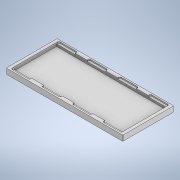
# Autodesk Inventor part: kbbottombodyethan
Saved by Autodesk Inventor 2021 (Build 250183000, 183)
## iProperties
Created: 2023-05-21
Part Number: kbbottombodyethan
Material: Generic
Document SubType Name: Modeling
Designer: ryand
Density: 1 g/cm^3
Appearance: Default
Author: ryand
Autodesk Inventor part; units mm, degrees
ref_plane "YZ Plane" through (0, 0, 0) normal (1, 0, 0) x (0, 1, 0)
ref_plane "XZ Plane" through (0, 0, 0) normal (0, 1, 0) x (-1, 0, 0)
ref_plane "XY Plane" through (0, 0, 0) normal (0, 0, 1) x (1, 0, 0)
sketch "Sketch1" plane through (0, 0, 0) normal (0, 1, 0) x (-1, 0, 0)
  line L0 (183.8315, -67.9127) -> (183.8315, 67.9127) construction
  line L1 (-179.8315, 79.4127) -> (-126.5543, 79.4127) construction
  line L2 (-122.5543, 75.4127) -> (-122.5543, 71.9127) construction
  line L3 (-81.7029, 71.9127) -> (-81.7029, 75.4127) construction
  line L4 (-77.7029, 79.4127) -> (-24.4257, 79.4127) construction
  line L5 (-20.4257, 75.4127) -> (-20.4257, 71.9127) construction
  line L6 (20.4257, 71.9127) -> (20.4257, 75.4127) construction
  line L7 (24.4257, 79.4127) -> (77.7029, 79.4127) construction
  line L8 (81.7029, 75.4127) -> (81.7029, 71.9127) construction
  line L9 (122.5543, 71.9127) -> (122.5543, 75.4127) construction
  line L10 (126.5543, 79.4127) -> (179.8315, 79.4127) construction
  line L11 (183.8315, 75.4127) -> (183.8315, 71.9127) construction
  line L12 (-126.5543, -79.4127) -> (-179.8315, -79.4127) construction
  line L13 (-183.8315, -75.4127) -> (-183.8315, -71.9127) construction
  line L14 (-122.5543, -71.9127) -> (-122.5543, -75.4127) construction
  line L15 (-81.7029, -75.4127) -> (-81.7029, -71.9127) construction
  line L16 (-24.4257, -79.4127) -> (-77.7029, -79.4127) construction
  line L17 (-20.4257, -71.9127) -> (-20.4257, -75.4127) construction
  line L18 (20.4257, -75.4127) -> (20.4257, -71.9127) construction
  line L19 (77.7029, -79.4127) -> (24.4257, -79.4127) construction
  line L20 (81.7029, -71.9127) -> (81.7029, -75.4127) construction
  line L21 (122.5543, -75.4127) -> (122.5543, -71.9127) construction
  line L22 (179.8315, -79.4127) -> (126.5543, -79.4127) construction
  line L23 (183.8315, -71.9127) -> (183.8315, -75.4127) construction
  line L24 (-122.5543, -71.9127) -> (-81.7029, -71.9127) construction
  line L25 (-20.4257, -71.9127) -> (20.4257, -71.9127) construction
  line L26 (81.7029, -71.9127) -> (122.5543, -71.9127) construction
  arc A0 (-183.8315, -75.4127) -> (-179.8315, -79.4127) centre (-179.8315, -75.4127) ccw construction
  arc A1 (-126.5543, -79.4127) -> (-122.5543, -75.4127) centre (-126.5543, -75.4127) ccw construction
  arc A2 (-81.7029, -75.4127) -> (-77.7029, -79.4127) centre (-77.7029, -75.4127) ccw construction
  arc A3 (-24.4257, -79.4127) -> (-20.4257, -75.4127) centre (-24.4257, -75.4127) ccw construction
  arc A4 (20.4257, -75.4127) -> (24.4257, -79.4127) centre (24.4257, -75.4127) ccw construction
  arc A5 (77.7029, -79.4127) -> (81.7029, -75.4127) centre (77.7029, -75.4127) ccw construction
  arc A6 (122.5543, -75.4127) -> (126.5543, -79.4127) centre (126.5543, -75.4127) ccw construction
  arc A7 (179.8315, -79.4127) -> (183.8315, -75.4127) centre (179.8315, -75.4127) ccw construction
  line L27 (183.8315, -67.9127) -> (183.8315, -71.9127) construction
  arc A8 (-179.8315, 79.4127) -> (-183.8315, 75.4127) centre (-179.8315, 75.4127) ccw construction
  arc A9 (-122.5543, 75.4127) -> (-126.5543, 79.4127) centre (-126.5543, 75.4127) ccw construction
  line L28 (-81.7029, 71.9127) -> (-122.5543, 71.9127) construction
  line L29 (20.4257, 71.9127) -> (-20.4257, 71.9127) construction
  line L30 (122.5543, 71.9127) -> (81.7029, 71.9127) construction
  line L31 (183.8315, 71.9127) -> (183.8315, 67.9127) construction
  arc A10 (-77.7029, 79.4127) -> (-81.7029, 75.4127) centre (-77.7029, 75.4127) ccw construction
  arc A11 (-20.4257, 75.4127) -> (-24.4257, 79.4127) centre (-24.4257, 75.4127) ccw construction
  arc A12 (24.4257, 79.4127) -> (20.4257, 75.4127) centre (24.4257, 75.4127) ccw construction
  arc A13 (81.7029, 75.4127) -> (77.7029, 79.4127) centre (77.7029, 75.4127) ccw construction
  arc A14 (126.5543, 79.4127) -> (122.5543, 75.4127) centre (126.5543, 75.4127) ccw construction
  arc A15 (183.8315, 75.4127) -> (179.8315, 79.4127) centre (179.8315, 75.4127) ccw construction
  line L32 (-183.8315, 75.4127) -> (-183.8315, -71.9127) construction
  line L33 (-126.5543, 79.9127) -> (-179.8315, 79.9127)
  arc A16 (-179.8315, 79.9127) -> (-184.3315, 75.4127) centre (-179.8315, 75.4127) ccw
  line L34 (-184.3315, 75.4127) -> (-184.3315, -71.9127)
  line L35 (-184.3315, -71.9127) -> (-184.3315, -75.4127)
  arc A17 (-184.3315, -75.4127) -> (-179.8315, -79.9127) centre (-179.8315, -75.4127) ccw
  line L36 (-179.8315, -79.9127) -> (-126.5543, -79.9127)
  arc A18 (-126.5543, -79.9127) -> (-122.0543, -75.4127) centre (-126.5543, -75.4127) ccw
  line L37 (-122.0543, -75.4127) -> (-122.0543, -72.4127)
  line L38 (-122.0543, -72.4127) -> (-82.2029, -72.4127)
  line L39 (-82.2029, -72.4127) -> (-82.2029, -75.4127)
  arc A19 (-82.2029, -75.4127) -> (-77.7029, -79.9127) centre (-77.7029, -75.4127) ccw
  line L40 (-77.7029, -79.9127) -> (-24.4257, -79.9127)
  arc A20 (-24.4257, -79.9127) -> (-19.9257, -75.4127) centre (-24.4257, -75.4127) ccw
  line L41 (-19.9257, -75.4127) -> (-19.9257, -72.4127)
  line L42 (-19.9257, -72.4127) -> (19.9257, -72.4127)
  line L43 (19.9257, -72.4127) -> (19.9257, -75.4127)
  arc A21 (19.9257, -75.4127) -> (24.4257, -79.9127) centre (24.4257, -75.4127) ccw
  line L44 (24.4257, -79.9127) -> (77.7029, -79.9127)
  arc A22 (77.7029, -79.9127) -> (82.2029, -75.4127) centre (77.7029, -75.4127) ccw
  line L45 (82.2029, -75.4127) -> (82.2029, -72.4127)
  line L46 (82.2029, -72.4127) -> (122.0543, -72.4127)
  line L47 (122.0543, -72.4127) -> (122.0543, -75.4127)
  arc A23 (122.0543, -75.4127) -> (126.5543, -79.9127) centre (126.5543, -75.4127) ccw
  line L48 (126.5543, -79.9127) -> (179.8315, -79.9127)
  arc A24 (179.8315, -79.9127) -> (184.3315, -75.4127) centre (179.8315, -75.4127) ccw
  line L49 (184.3315, -75.4127) -> (184.3315, -71.9127)
  line L50 (184.3315, -71.9127) -> (184.3315, -67.9127)
  line L51 (184.3315, -67.9127) -> (184.3315, 67.9127)
  line L52 (184.3315, 67.9127) -> (184.3315, 71.9127)
  line L53 (184.3315, 71.9127) -> (184.3315, 75.4127)
  arc A25 (184.3315, 75.4127) -> (179.8315, 79.9127) centre (179.8315, 75.4127) ccw
  line L54 (179.8315, 79.9127) -> (126.5543, 79.9127)
  arc A26 (126.5543, 79.9127) -> (122.0543, 75.4127) centre (126.5543, 75.4127) ccw
  line L55 (122.0543, 75.4127) -> (122.0543, 72.4127)
  line L56 (122.0543, 72.4127) -> (82.2029, 72.4127)
  line L57 (82.2029, 72.4127) -> (82.2029, 75.4127)
  arc A27 (82.2029, 75.4127) -> (77.7029, 79.9127) centre (77.7029, 75.4127) ccw
  line L58 (77.7029, 79.9127) -> (24.4257, 79.9127)
  arc A28 (24.4257, 79.9127) -> (19.9257, 75.4127) centre (24.4257, 75.4127) ccw
  line L59 (19.9257, 75.4127) -> (19.9257, 72.4127)
  line L60 (19.9257, 72.4127) -> (-19.9257, 72.4127)
  line L61 (-19.9257, 72.4127) -> (-19.9257, 75.4127)
  arc A29 (-19.9257, 75.4127) -> (-24.4257, 79.9127) centre (-24.4257, 75.4127) ccw
  line L62 (-24.4257, 79.9127) -> (-77.7029, 79.9127)
  arc A30 (-77.7029, 79.9127) -> (-82.2029, 75.4127) centre (-77.7029, 75.4127) ccw
  line L63 (-82.2029, 75.4127) -> (-82.2029, 72.4127)
  line L64 (-82.2029, 72.4127) -> (-122.0543, 72.4127)
  line L65 (-122.0543, 72.4127) -> (-122.0543, 75.4127)
  arc A31 (-122.0543, 75.4127) -> (-126.5543, 79.9127) centre (-126.5543, 75.4127) ccw
  line L66 (-179.8315, 75.4127) -> (179.8315, -75.4127) construction
  line L67 (179.8315, 75.4127) -> (-179.8315, -75.4127) construction
  line L68 (-192.3315, 84.9127) -> (192.3315, 84.9127)
  line L69 (194.3315, 82.9127) -> (194.3315, -82.9127)
  line L70 (192.3315, -84.9127) -> (-192.3315, -84.9127)
  line L71 (-194.3315, -82.9127) -> (-194.3315, 82.9127)
  line L72 (-194.3315, 84.9127) -> (194.3315, -84.9127) construction
  line L73 (194.3315, 84.9127) -> (-194.3315, -84.9127) construction
  arc A32 (-192.3315, 84.9127) -> (-194.3315, 82.9127) centre (-192.3315, 82.9127) ccw
  arc A33 (194.3315, 82.9127) -> (192.3315, 84.9127) centre (192.3315, 82.9127) ccw
  arc A34 (192.3315, -84.9127) -> (194.3315, -82.9127) centre (192.3315, -82.9127) ccw
  arc A35 (-194.3315, -82.9127) -> (-192.3315, -84.9127) centre (-192.3315, -82.9127) ccw
  point P0 (0, 0)
  point P1 (0, 0)
  dimension "d9" = 4
  dimension "d10" = 4
  dimension "d11" = 4
  dimension "d12" = 4
  dimension "d13" = 0.5
  dimension "d16" = 159.8253
  dimension "d17" = 368.6629
  dimension "d18" = 388.6629
  dimension "d19" = 169.8253
  dimension "d20" = 2
  constraints: 148 end point, 72 point on circle, 39 tangent, 36 centre point, 22 parallel, 15 equal radius, 8 point on line, 5 horizontal, 3 midpoint, 3 perpendicular, 2 collinear, 2 vertical, 49 other
  measures "d9" radius of A0
  measures "d10" radius of A2
  measures "d11" radius of A8
  measures "d12" radius of A10
  measures "d13" distance between parallel lines of L1 L33
  measures "d16" distance between parallel lines of L36 L33
  measures "d17" distance between parallel lines of L51 L34
  measures "d18" distance of L72.end L73.end
  measures "d19" distance of L73.start L72.end
  measures "d20" radius of A32
extrude "Extrusion1" add sketch "Sketch1" against normal blind 4
sketch "Sketch2" plane through (0, -4, 0) normal (0, -1, 0) x (1, 0, 0)
  line L0 (-192.3315, -84.9127) -> (192.3315, -84.9127) projected
  arc A0 (192.3315, -84.9127) -> (194.3315, -82.9127) centre (192.3315, -82.9127) ccw projected
  line L1 (194.3315, -82.9127) -> (194.3315, 82.9127) projected
  arc A1 (194.3315, 82.9127) -> (192.3315, 84.9127) centre (192.3315, 82.9127) ccw projected
  line L2 (192.3315, 84.9127) -> (-192.3315, 84.9127) projected
  arc A2 (-192.3315, 84.9127) -> (-194.3315, 82.9127) centre (-192.3315, 82.9127) ccw projected
  line L3 (-194.3315, 82.9127) -> (-194.3315, -82.9127) projected
  arc A3 (-194.3315, -82.9127) -> (-192.3315, -84.9127) centre (-192.3315, -82.9127) ccw projected
  arc A4 (126.5543, 79.9127) -> (122.0543, 75.4127) centre (126.5543, 75.4127) ccw projected
  line L4 (126.5543, 79.9127) -> (179.8315, 79.9127) projected
  arc A5 (184.3315, 75.4127) -> (179.8315, 79.9127) centre (179.8315, 75.4127) ccw projected
  line L5 (184.3315, 75.4127) -> (184.3315, -75.4127) projected
  arc A6 (179.8315, -79.9127) -> (184.3315, -75.4127) centre (179.8315, -75.4127) ccw projected
  line L6 (179.8315, -79.9127) -> (126.5543, -79.9127) projected
  arc A7 (122.0543, -75.4127) -> (126.5543, -79.9127) centre (126.5543, -75.4127) ccw projected
  line L7 (122.0543, -75.4127) -> (122.0543, -72.4127) projected
  line L8 (122.0543, -72.4127) -> (82.2029, -72.4127) projected
  line L9 (82.2029, -72.4127) -> (82.2029, -75.4127) projected
  arc A8 (77.7029, -79.9127) -> (82.2029, -75.4127) centre (77.7029, -75.4127) ccw projected
  line L10 (77.7029, -79.9127) -> (24.4257, -79.9127) projected
  arc A9 (19.9257, -75.4127) -> (24.4257, -79.9127) centre (24.4257, -75.4127) ccw projected
  line L11 (19.9257, -75.4127) -> (19.9257, -72.4127) projected
  line L12 (19.9257, -72.4127) -> (-19.9257, -72.4127) projected
  line L13 (-19.9257, -72.4127) -> (-19.9257, -75.4127) projected
  arc A10 (-24.4257, -79.9127) -> (-19.9257, -75.4127) centre (-24.4257, -75.4127) ccw projected
  line L14 (-24.4257, -79.9127) -> (-77.7029, -79.9127) projected
  arc A11 (-82.2029, -75.4127) -> (-77.7029, -79.9127) centre (-77.7029, -75.4127) ccw projected
  line L15 (-82.2029, -75.4127) -> (-82.2029, -72.4127) projected
  line L16 (-82.2029, -72.4127) -> (-122.0543, -72.4127) projected
  line L17 (-122.0543, -72.4127) -> (-122.0543, -75.4127) projected
  arc A12 (-126.5543, -79.9127) -> (-122.0543, -75.4127) centre (-126.5543, -75.4127) ccw projected
  line L18 (-126.5543, -79.9127) -> (-179.8315, -79.9127) projected
  arc A13 (-184.3315, -75.4127) -> (-179.8315, -79.9127) centre (-179.8315, -75.4127) ccw projected
  line L19 (-184.3315, -75.4127) -> (-184.3315, 75.4127) projected
  arc A14 (-179.8315, 79.9127) -> (-184.3315, 75.4127) centre (-179.8315, 75.4127) ccw projected
  line L20 (-179.8315, 79.9127) -> (-126.5543, 79.9127) projected
  arc A15 (-122.0543, 75.4127) -> (-126.5543, 79.9127) centre (-126.5543, 75.4127) ccw projected
  line L21 (-122.0543, 75.4127) -> (-122.0543, 72.4127) projected
  line L22 (-122.0543, 72.4127) -> (-82.2029, 72.4127) projected
  line L23 (-82.2029, 72.4127) -> (-82.2029, 75.4127) projected
  arc A16 (-77.7029, 79.9127) -> (-82.2029, 75.4127) centre (-77.7029, 75.4127) ccw projected
  line L24 (-77.7029, 79.9127) -> (-24.4257, 79.9127) projected
  arc A17 (-19.9257, 75.4127) -> (-24.4257, 79.9127) centre (-24.4257, 75.4127) ccw projected
  line L25 (-19.9257, 75.4127) -> (-19.9257, 72.4127) projected
  line L26 (-19.9257, 72.4127) -> (19.9257, 72.4127) projected
  line L27 (19.9257, 72.4127) -> (19.9257, 75.4127) projected
  arc A18 (24.4257, 79.9127) -> (19.9257, 75.4127) centre (24.4257, 75.4127) ccw projected
  line L28 (24.4257, 79.9127) -> (77.7029, 79.9127) projected
  arc A19 (82.2029, 75.4127) -> (77.7029, 79.9127) centre (77.7029, 75.4127) ccw projected
  line L29 (82.2029, 75.4127) -> (82.2029, 72.4127) projected
  line L30 (82.2029, 72.4127) -> (122.0543, 72.4127) projected
  line L31 (122.0543, 72.4127) -> (122.0543, 75.4127) projected
  line L32 (-184.3315, -75.4127) -> (-184.3315, 75.4127) projected
  line L33 (184.3315, 75.4127) -> (184.3315, -75.4127) projected
  line L34 (-184.3315, 72.4127) -> (184.3315, 72.4127)
  line L35 (184.3315, 72.4127) -> (184.3315, -72.4127)
  line L36 (184.3315, -72.4127) -> (-184.3315, -72.4127)
  line L37 (-184.3315, -72.4127) -> (-184.3315, 72.4127)
  point P0 (0, 0)
  constraints: 8 end point, 2 parallel, 2 point on line, 1 horizontal, 1 perpendicular
extrude "Extrusion2" add sketch "Sketch2" along normal blind 7 contours A3 L3 A2 L2 A1 L1 A0 L0 | L4 A5 L5 L34 L31 A4 | L34 L27 A18 L28 A19 L29 | L5 A6 L6 A7 L7 L36 | L34 L23 A16 L24 A17 L25 | L9 A8 L10 A9 L11 L36 | L34 L19 A14 L20 A15 L21 | L13 A10 L14 A11 L15 L36 | L36 L17 A12 L18 A13 L19
sketch "Sketch3" plane through (0, -11, 0) normal (0, -1, 0) x (1, 0, 0)
  arc A0 (192.3315, -84.9127) -> (194.3315, -82.9127) centre (192.3315, -82.9127) ccw projected
  line L0 (194.3315, -82.9127) -> (194.3315, 82.9127) projected
  arc A1 (194.3315, 82.9127) -> (192.3315, 84.9127) centre (192.3315, 82.9127) ccw projected
  line L1 (192.3315, 84.9127) -> (-192.3315, 84.9127) projected
  arc A2 (-192.3315, 84.9127) -> (-194.3315, 82.9127) centre (-192.3315, 82.9127) ccw projected
  line L2 (-194.3315, 82.9127) -> (-194.3315, -82.9127) projected
  arc A3 (-194.3315, -82.9127) -> (-192.3315, -84.9127) centre (-192.3315, -82.9127) ccw projected
  line L3 (-192.3315, -84.9127) -> (192.3315, -84.9127) projected
  line L4 (184.3315, 72.4127) -> (184.3315, -72.4127) projected
  line L5 (184.3315, -72.4127) -> (-184.3315, -72.4127) projected
  line L6 (-184.3315, -72.4127) -> (-184.3315, 72.4127) projected
  line L7 (-184.3315, 72.4127) -> (184.3315, 72.4127) projected
  point P0 (0, 0)
extrude "Extrusion3" add sketch "Sketch3" along normal blind 7 contours L3 A3 L2 A2 L1 A1 L0 A0 | L4 L5 L6 L7
body "Solid1"
